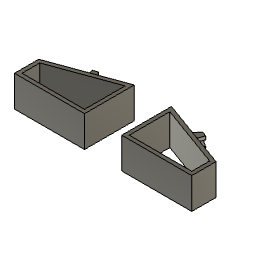
Microfreak Parametric v15 v9 (Autodesk Fusion 360 design; units mm, degrees)
Autodesk Fusion 360 part; units mm, degrees
note: some values were not read from the file. Set by a fixed rule: which sketch regions a step uses.
sketch "StandBase" plane through (0, 0, 0) normal (0, 0, 1) x (1, 0, 0)
  line L0 (0, 0) -> (112.7631, 0)
  line L1 (112.7631, 0) -> (112.7631, 80)
  line L2 (112.7631, 80) -> (0, 38.9576)
  line L3 (0, 0) -> (0, 38.9576)
  line L4 (6, 6) -> (6, 34.7563)
  line L5 (106.7631, 71.4311) -> (6, 34.7563)
  line L6 (106.7631, 6) -> (106.7631, 71.4311)
  line L7 (6, 6) -> (106.7631, 6)
  dimension "d12" = 80
  dimension "d13" = 70
  dimension "d15" = 120
  constraint coincident L0.start L3.start
  constraint horizontal L0
  constraint perpendicular L0 L1
  constraint perpendicular L0 L3
  measures "d12" distance of L0.end L1.end
  measures "d13" angle of L1 L2
  measures "d15" distance of L1.end L2.end
extrude "Extrude1" add sketch "StandBase" along normal blind 50 makes body 1
ref_plane "WorkPlane1" through (56.3816, 40, 25) normal (0, 0, -1) x (-1, 0, 0)
sketch "MicrofreakTab" plane through (56.3816, 50, 25) normal (0, 0, -1) x (1, 0, 0)
  line L0 (0, -9.4788) -> (13.1557, -14.2671)
  line L1 (0, -9.4788) -> (-5.1303, -23.5742)
  line L2 (-5.1303, -23.5742) -> (2.3872, -26.3103)
  line L3 (2.3872, -26.3103) -> (13.1557, -14.2671)
  line L4 (56.3816, -30) -> (-56.3816, 11.0424)
  dimension "d51" = 14
  dimension "d62" = 15
  dimension "d63" = 8
  constraint perpendicular L0 L1
  constraint perpendicular L1 L2
  constraint collinear L0 L4
  constraint midpoint L0.start L4
  measures "d51" distance of L0.start L0.end
  measures "d62" distance of L0.start L1.end
  measures "d63" distance of L1.end L2.end
extrude "Extrude6" add sketch "MicrofreakTab" along normal blind 16.5 from surface at 1.5 bodies 1
mirror "Mirror4" about plane through (56.3816, 40, 25) normal (0, 0, -1) of "Extrude6"
ref_plane "WorkPlane8" through (56.3816, 59.4788, 25) normal (-0.34202, 0.939693, 0) x (-0.939693, -0.34202, 0)
sketch "MicrofreakTab Hole" plane through (56.3816, 59.4788, 25) normal (-0.34202, 0.939693, 0) x (-0.939693, -0.34202, 0)
  line L0 (0, 1.5) -> (0, 7.9863)
  circle A0 centre (0, 7.9863) radius 4.5
  line L1 (0, 1.5) -> (0, 18)
  point P0 (-14, 1.5)
  point P1 (0, 1.5)
  dimension "d59" = 9
  constraint coincident L0.end A0.centre
  constraint coincident L0.start L1.start
  constraint collinear L0 L1
  measures "d59" diameter of A0
extrude "Extrude8" cut sketch "MicrofreakTab Hole" along normal blind 15 bodies 1
ref_plane "WorkPlane10" through (142.7631, 40, 25) normal (1, 0, 0) x (0, 1, 0)
mirror "Mirror5" about plane through (142.7631, 40, 25) normal (1, 0, 0) of bodies 1 makes body 2
equation "tabHeight = 15 mm" comment "Should not edit this parameter"
equation "tabTopLength = 8 mm" comment "Should not edit this parameter"
equation "tabBottomLength = 14 mm" comment "Should not edit this parameter"
equation "tabSpacer = 3 mm" comment "Should not edit this parameter"
equation "tabCircleRadius = 4.5 mm" comment "Should not edit this parameter"
equation "tabCircleSpacer = 5 mm" comment "Should not edit this parameter"
equation "tilt = 20 deg" comment "Device tilt"
equation "baseWidth = 50 mm" comment "Stand width"
equation "baseHeight = 80 mm" comment "Stand height"
equation "thickness = 6 mm" comment "Stand thickness"
equation "roundness = 1 mm" comment "Stand roundness"
equation "d12 = baseHeight"
equation "d13 = 90 deg - tilt"
equation "baseLength = 120 mm" comment "Stand length"
equation "d15 = baseLength"
equation "d16 = -thickness"
equation "d17 = baseWidth"
equation "tabWidth = 16.5 mm" comment "Should not edit this parameter"
equation "d51 = tabBottomLength"
equation "d52 = tabSpacer / 2"
equation "d53 = tabWidth"
equation "d59 = tabCircleRadius * 2"
equation "d62 = tabHeight"
equation "d63 = tabTopLength"
equation "d64 = tabHeight"
equation "d66 = tabHeight * 2"
named bodies: "Left Leg", "Right Leg"
